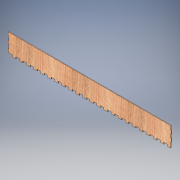
# Autodesk Inventor part: КВ33.044.004 - Стенка блока управления
Saved by Autodesk Inventor 2019 (Build 230136000, 136)
## iProperties
Created: 2019-08-10
Part Number: КВ33.044.004 - Стенка блока управления
Material: Дерево (береза)
Document SubType Name: Modeling
Designer: Петров Иван
Density: 0.55 g/cm^3
Appearance: Береза — натуральный — полированный
Author: Петров Иван
Autodesk Inventor part; units mm, degrees
ref_plane "YZ Plane" through (0, 0, 0) normal (1, 0, 0) x (0, 1, 0)
ref_plane "XZ Plane" through (0, 0, 0) normal (0, 1, 0) x (-1, 0, 0)
ref_plane "XY Plane" through (0, 0, 0) normal (0, 0, 1) x (1, 0, 0)
sketch "Эскиз1" plane through (0, 0, 0) normal (0, 0, 1) x (1, 0, 0)
  line L0 (-367, -44.25) -> (367, -44.25)
  line L1 (367, -44.25) -> (367, 44.25)
  line L2 (367, 44.25) -> (-367, 44.25)
  line L3 (-367, 44.25) -> (-367, -44.25)
  line L4 (-367, -44.25) -> (367, 44.25) construction
  line L5 (367, -44.25) -> (-367, 44.25) construction
  point P0 (0, 0)
  dimension "d0" = 734
  dimension "d1" = 88.5
  constraints: 12 end point, 2 midpoint, 2 parallel, 1 horizontal, 1 perpendicular
  measures "d0" distance of L2.end L1.end
  measures "d1" distance of L1.end L0.end
extrude "Выдавливание1" add sketch "Эскиз1" along normal blind 3
sketch "Эскиз2" plane through (0, 0, 3) normal (0, 0, 1) x (1, 0, 0)
  line L0 (-367, -44.25) -> (367, -44.25) projected
  line L1 (-367, -44.25) -> (-351, -44.25)
  line L2 (-351, -44.25) -> (-351, -36.25)
  line L3 (-351, -36.25) -> (-367, -36.25)
  line L4 (-367, -36.25) -> (-367, -44.25)
  line L5 (-335, -44.25) -> (-319, -44.25)
  line L6 (-319, -44.25) -> (-319, -36.25)
  line L7 (-319, -36.25) -> (-335, -36.25)
  line L8 (-335, -36.25) -> (-335, -44.25)
  line L9 (-303, -44.25) -> (-287, -44.25)
  line L10 (-287, -44.25) -> (-287, -36.25)
  line L11 (-287, -36.25) -> (-303, -36.25)
  line L12 (-303, -36.25) -> (-303, -44.25)
  line L13 (-271, -44.25) -> (-255, -44.25)
  line L14 (-255, -44.25) -> (-255, -36.25)
  line L15 (-255, -36.25) -> (-271, -36.25)
  line L16 (-271, -36.25) -> (-271, -44.25)
  line L17 (-239, -44.25) -> (-223, -44.25)
  line L18 (-223, -44.25) -> (-223, -36.25)
  line L19 (-223, -36.25) -> (-239, -36.25)
  line L20 (-239, -36.25) -> (-239, -44.25)
  line L21 (-207, -44.25) -> (-191, -44.25)
  line L22 (-191, -44.25) -> (-191, -36.25)
  line L23 (-191, -36.25) -> (-207, -36.25)
  line L24 (-207, -36.25) -> (-207, -44.25)
  line L25 (-175, -44.25) -> (-159, -44.25)
  line L26 (-159, -44.25) -> (-159, -36.25)
  line L27 (-159, -36.25) -> (-175, -36.25)
  line L28 (-175, -36.25) -> (-175, -44.25)
  line L29 (-143, -44.25) -> (-127, -44.25)
  line L30 (-127, -44.25) -> (-127, -36.25)
  line L31 (-127, -36.25) -> (-143, -36.25)
  line L32 (-143, -36.25) -> (-143, -44.25)
  line L33 (-111, -44.25) -> (-95, -44.25)
  line L34 (-95, -44.25) -> (-95, -36.25)
  line L35 (-95, -36.25) -> (-111, -36.25)
  line L36 (-111, -36.25) -> (-111, -44.25)
  line L37 (-79, -44.25) -> (-63, -44.25)
  line L38 (-63, -44.25) -> (-63, -36.25)
  line L39 (-63, -36.25) -> (-79, -36.25)
  line L40 (-79, -36.25) -> (-79, -44.25)
  line L41 (-47, -44.25) -> (-31, -44.25)
  line L42 (-31, -44.25) -> (-31, -36.25)
  line L43 (-31, -36.25) -> (-47, -36.25)
  line L44 (-47, -36.25) -> (-47, -44.25)
  line L45 (-15, -44.25) -> (1, -44.25)
  line L46 (1, -44.25) -> (1, -36.25)
  line L47 (1, -36.25) -> (-15, -36.25)
  line L48 (-15, -36.25) -> (-15, -44.25)
  line L49 (17, -44.25) -> (33, -44.25)
  line L50 (33, -44.25) -> (33, -36.25)
  line L51 (33, -36.25) -> (17, -36.25)
  line L52 (17, -36.25) -> (17, -44.25)
  line L53 (49, -44.25) -> (65, -44.25)
  line L54 (65, -44.25) -> (65, -36.25)
  line L55 (65, -36.25) -> (49, -36.25)
  line L56 (49, -36.25) -> (49, -44.25)
  line L57 (81, -44.25) -> (97, -44.25)
  line L58 (97, -44.25) -> (97, -36.25)
  line L59 (97, -36.25) -> (81, -36.25)
  line L60 (81, -36.25) -> (81, -44.25)
  line L61 (113, -44.25) -> (129, -44.25)
  line L62 (129, -44.25) -> (129, -36.25)
  line L63 (129, -36.25) -> (113, -36.25)
  line L64 (113, -36.25) -> (113, -44.25)
  line L65 (145, -44.25) -> (161, -44.25)
  line L66 (161, -44.25) -> (161, -36.25)
  line L67 (161, -36.25) -> (145, -36.25)
  line L68 (145, -36.25) -> (145, -44.25)
  line L69 (177, -44.25) -> (193, -44.25)
  line L70 (193, -44.25) -> (193, -36.25)
  line L71 (193, -36.25) -> (177, -36.25)
  line L72 (177, -36.25) -> (177, -44.25)
  line L73 (209, -44.25) -> (225, -44.25)
  line L74 (225, -44.25) -> (225, -36.25)
  line L75 (225, -36.25) -> (209, -36.25)
  line L76 (209, -36.25) -> (209, -44.25)
  line L77 (241, -44.25) -> (257, -44.25)
  line L78 (257, -44.25) -> (257, -36.25)
  line L79 (257, -36.25) -> (241, -36.25)
  line L80 (241, -36.25) -> (241, -44.25)
  line L81 (273, -44.25) -> (289, -44.25)
  line L82 (289, -44.25) -> (289, -36.25)
  line L83 (289, -36.25) -> (273, -36.25)
  line L84 (273, -36.25) -> (273, -44.25)
  line L85 (305, -44.25) -> (321, -44.25)
  line L86 (321, -44.25) -> (321, -36.25)
  line L87 (321, -36.25) -> (305, -36.25)
  line L88 (305, -36.25) -> (305, -44.25)
  line L89 (337, -44.25) -> (353, -44.25)
  line L90 (353, -44.25) -> (353, -36.25)
  line L91 (353, -36.25) -> (337, -36.25)
  line L92 (337, -36.25) -> (337, -44.25)
  point P0 (0, 0)
  dimension "d4" = 16
  dimension "d5" = 8
  dimension "d8" = 32
  constraints: 184 end point, 2 horizontal, 2 parallel, 1 perpendicular, 176 other
  measures "d4" distance of L3.end L2.end
  measures "d5" distance of L2.end L1.end
  measures "d8" distance of L2.end L6.end
extrude "Выдавливание2" cut sketch "Эскиз2" against normal blind 3
sketch "Эскиз3" plane through (0, 0, 3) normal (0, 0, 1) x (1, 0, 0)
  line L0 (367, 44.25) -> (-367, 44.25) projected
  line L1 (-367, 44.25) -> (-370, 44.25)
  line L2 (-370, 44.25) -> (-370, 28.25)
  line L3 (-370, 28.25) -> (-367, 28.25)
  line L4 (-367, 28.25) -> (-367, 44.25)
  line L5 (-367, 12.25) -> (-370, 12.25)
  line L6 (-370, 12.25) -> (-370, -3.75)
  line L7 (-370, -3.75) -> (-367, -3.75)
  line L8 (-367, -3.75) -> (-367, 12.25)
  line L9 (-367, -19.75) -> (-370, -19.75)
  line L10 (-370, -19.75) -> (-370, -35.75)
  line L11 (-370, -35.75) -> (-367, -35.75)
  line L12 (-367, -35.75) -> (-367, -19.75)
  line L13 (367, -44.25) -> (367, 44.25) projected
  line L14 (367, 28.25) -> (367, 44.25)
  line L15 (367, 28.25) -> (370, 28.25)
  line L16 (370, 28.25) -> (370, 12.25)
  line L17 (370, 12.25) -> (367, 12.25)
  line L18 (367, 12.25) -> (367, 28.25)
  line L19 (370, -19.75) -> (367, -19.75)
  line L20 (370, -3.75) -> (370, -19.75)
  line L21 (367, -3.75) -> (370, -3.75)
  line L22 (367, -19.75) -> (367, -3.75)
  point P0 (0, 0)
  dimension "d15" = 3
  dimension "d16" = 16
  dimension "d19" = 32
  dimension "d24" = 3
  dimension "d25" = 16
  dimension "d28" = 32
  constraints: 42 end point, 4 parallel, 2 collinear, 2 horizontal, 2 perpendicular, 2 vertical, 1 point on line, 23 other
  measures "d15" distance of L3.end L2.end
  measures "d16" distance of L2.end L1.end
  measures "d19" distance of L2.end L6.end
  measures "d24" distance of L16.end L17.end
  measures "d25" distance of L15.end L16.end
  measures "d28" distance of L16.end L19.start
extrude "Выдавливание3" add sketch "Эскиз3" against normal blind 3
